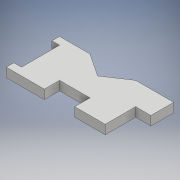
# Autodesk Inventor part: P2-3
Saved by Autodesk Inventor 2017 (Build 210142000, 142)
## iProperties
Created: 2017-02-09
Part Number: P2-3
Material: Generic
Document SubType Name: Modeling
Designer: Schaffel
Density: 1 g/cm^3
Appearance: Default
Author: Schaffel
Autodesk Inventor part; units mm, degrees
ref_plane "YZ Plane" through (0, 0, 0) normal (1, 0, 0) x (0, 1, 0)
ref_plane "XZ Plane" through (0, 0, 0) normal (0, 1, 0) x (-1, 0, 0)
ref_plane "XY Plane" through (0, 0, 0) normal (0, 0, 1) x (1, 0, 0)
sketch "Sketch1" plane through (0, 0, 0) normal (0, 0, 1) x (1, 0, 0)
  line L0 (0, 0) -> (50, 0)
  line L1 (50, 0) -> (50, 20)
  line L2 (50, 20) -> (90, 20)
  line L3 (90, 20) -> (90, 0)
  line L4 (90, 0) -> (130, 0)
  line L5 (130, 0) -> (130, 40)
  line L6 (130, 40) -> (150, 40)
  line L7 (150, 40) -> (150, 70)
  line L8 (150, 70) -> (100, 70)
  line L9 (70, 50) -> (100, 70)
  line L10 (40, 70) -> (70, 50)
  line L11 (40, 70) -> (0, 70)
  line L12 (0, 70) -> (0, 60)
  line L13 (0, 60) -> (10, 60)
  line L14 (10, 60) -> (10, 10)
  line L15 (10, 10) -> (0, 10)
  line L16 (0, 10) -> (0, 0)
  dimension "d0" = 50
  constraints: 34 end point, 11 perpendicular, 3 point on line, 1 horizontal
  measures "d0" distance of L0.start L0.end
extrude "Extrusion1" add sketch "Sketch1" along normal blind 12
body "Solid1"
